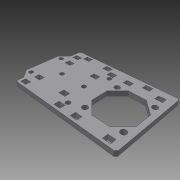
# Autodesk Inventor part: x_iddler_bottom
Saved by Autodesk Inventor 2014 (Build 180170000, 170)
## iProperties
Created: 2013-12-02
Part Number: x_iddler_bottom
Material: Generic
Document SubType Name: Modeling
Designer: buben
Density: 1 g/cm^3
Appearance: Default
Author: buben
Autodesk Inventor part; units mm, degrees
ref_plane "YZ Plane" through (0, 0, 0) normal (1, 0, 0) x (0, 1, 0)
ref_plane "XZ Plane" through (0, 0, 0) normal (0, 1, 0) x (-1, 0, 0)
ref_plane "XY Plane" through (0, 0, 0) normal (0, 0, 1) x (1, 0, 0)
sketch "Sketch1" plane through (0, 0, 0) normal (0, 0, 1) x (1, 0, 0)
  line L0 (0, 0) -> (-128, 0)
  line L1 (-128, 86) -> (0, 86)
  line L2 (0, 86) -> (0, 0)
  line L3 (-128, 71) -> (-138, 61)
  line L4 (-138, 61) -> (-138, 19)
  line L5 (-138, 19) -> (-128, 9)
  line L6 (-128, 0) -> (-128, 9)
  line L7 (-128, 71) -> (-128, 86)
  line L8 (-52, 9) -> (-44, 9)
  line L9 (-44, 9) -> (-44, 3)
  line L10 (-44, 3) -> (-52, 3)
  line L11 (-52, 3) -> (-52, 9)
  line L12 (-52, 77) -> (-44, 77)
  line L13 (-44, 77) -> (-44, 71)
  line L14 (-44, 71) -> (-52, 71)
  line L15 (-52, 71) -> (-52, 77)
  line L16 (-16, 77) -> (-8, 77)
  line L17 (-8, 77) -> (-8, 71)
  line L18 (-8, 71) -> (-16, 71)
  line L19 (-16, 71) -> (-16, 77)
  line L20 (-16, 9) -> (-8, 9)
  line L21 (-8, 9) -> (-8, 3)
  line L22 (-8, 3) -> (-16, 3)
  line L23 (-16, 3) -> (-16, 9)
  line L24 (-34, 83) -> (-26, 83)
  line L25 (-26, 83) -> (-26, 77)
  line L26 (-26, 77) -> (-34, 77)
  line L27 (-34, 77) -> (-34, 83)
  line L28 (-6, 49.9411) -> (-6, 30.0589)
  line L29 (-6, 30.0589) -> (-20.0589, 16)
  line L30 (-20.0589, 16) -> (-39.9411, 16)
  line L31 (-39.9411, 16) -> (-54, 30.0589)
  line L32 (-54, 30.0589) -> (-54, 49.9411)
  line L33 (-54, 49.9411) -> (-39.9411, 64)
  line L34 (-39.9411, 64) -> (-20.0589, 64)
  line L35 (-20.0589, 64) -> (-6, 49.9411)
  line L36 (-51, 61) -> (-9, 61) construction
  line L37 (-9, 61) -> (-9, 19) construction
  line L38 (-9, 19) -> (-51, 19) construction
  line L39 (-51, 19) -> (-51, 61) construction
  circle A0 centre (-51, 61) radius 3.2
  circle A1 centre (-51, 19) radius 3.2
  circle A2 centre (-9, 19) radius 3.2
  circle A3 centre (-9, 61) radius 3.2
  circle A4 centre (-131, 60) radius 2.75
  circle A5 centre (-131, 20) radius 2.75
  line L40 (-124, 77) -> (-116, 77)
  line L41 (-116, 77) -> (-116, 71)
  line L42 (-116, 71) -> (-124, 71)
  line L43 (-124, 71) -> (-124, 77)
  line L44 (-124, 9) -> (-116, 9)
  line L45 (-116, 9) -> (-116, 3)
  line L46 (-116, 3) -> (-124, 3)
  line L47 (-124, 3) -> (-124, 9)
  line L48 (-121, 63) -> (-113, 63)
  line L49 (-113, 63) -> (-113, 57)
  line L50 (-113, 57) -> (-121, 57)
  line L51 (-121, 57) -> (-121, 63)
  line L52 (-121, 23) -> (-113, 23)
  line L53 (-113, 23) -> (-113, 17)
  line L54 (-113, 17) -> (-121, 17)
  line L55 (-121, 17) -> (-121, 23)
  circle A6 centre (-66, 67) radius 2.75
  circle A7 centre (-66, 13) radius 2.75
  line L56 (-60, 86) -> (-60, 0) construction
  line L57 (-132, 67) -> (-60, 67) construction
  line L58 (-132, 13) -> (-60, 13) construction
  line L59 (-83, 63) -> (-75, 63)
  line L60 (-75, 63) -> (-75, 57)
  line L61 (-75, 57) -> (-83, 57)
  line L62 (-83, 57) -> (-83, 63)
  line L63 (-83, 23) -> (-75, 23)
  line L64 (-75, 23) -> (-75, 17)
  line L65 (-75, 17) -> (-83, 17)
  line L66 (-83, 17) -> (-83, 23)
  line L67 (-73, 77) -> (-65, 77)
  line L68 (-65, 77) -> (-65, 71)
  line L69 (-65, 71) -> (-73, 71)
  line L70 (-73, 71) -> (-73, 77)
  line L71 (-73, 9) -> (-65, 9)
  line L72 (-65, 9) -> (-65, 3)
  line L73 (-65, 3) -> (-73, 3)
  line L74 (-73, 3) -> (-73, 9)
  line L75 (-113, 83) -> (-105, 83)
  line L76 (-105, 83) -> (-105, 77)
  line L77 (-105, 77) -> (-113, 77)
  line L78 (-113, 77) -> (-113, 83)
  line L79 (-84, 83) -> (-76, 83)
  line L80 (-76, 83) -> (-76, 77)
  line L81 (-76, 77) -> (-84, 77)
  line L82 (-84, 77) -> (-84, 83)
  circle A8 centre (-106, 40) radius 2.75
  circle A9 centre (-74, 40) radius 2.75
  point P0 (-30, 40)
  point P1 (-138, 40)
  point P2 (-54, 40)
  point P3 (-51, 40)
  point P4 (-30, 61)
  point P5 (-30, 64)
  dimension "d1" = 45
  dimension "d2" = 10
  dimension "d3" = 6
  dimension "d4" = 6
  dimension "d5" = 3
  dimension "d6" = 8
  dimension "d7" = 8
  dimension "d8" = 6
  dimension "d10" = 3
  dimension "d11" = 48
  dimension "d12" = 8
  dimension "d13" = 6
  dimension "d14" = 42
  dimension "d15" = 42
  dimension "d16" = 6.4
  dimension "d17" = 6.4
  dimension "d18" = 6.4
  dimension "d19" = 6.4
  dimension "d20" = 5.5
  dimension "d21" = 5.5
  dimension "d22" = 7
  dimension "d23" = 11
  dimension "d24" = 11
  dimension "d25" = 6
  dimension "d26" = 8
  dimension "d27" = 6
  dimension "d28" = 6
  dimension "d29" = 8
  dimension "d30" = 6
  dimension "d31" = 8
  dimension "d32" = 8
  dimension "d33" = 5.5
  dimension "d34" = 5.5
  dimension "d35" = 4
  dimension "d36" = 4
  dimension "d37" = 8
  dimension "d38" = 8
  dimension "d39" = 8
  dimension "d40" = 4
  dimension "d41" = 8
  dimension "d42" = 128
  dimension "d43" = 68
  dimension "d44" = 8
  dimension "d45" = 43
  dimension "d47" = 10
  dimension "d48" = 15
  dimension "d49" = 62
  dimension "d50" = 10
  dimension "d52" = 8
  dimension "d53" = 3
  dimension "d54" = 8
  dimension "d55" = 3
  dimension "d56" = 5.5
  dimension "d57" = 5.5
  dimension "d58" = 14
  dimension "d59" = 32
  dimension "d65" = 34
  constraints: 166 end point, 37 parallel, 29 collinear, 21 perpendicular, 17 horizontal, 10 centre point, 9 horizontal alignment, 8 point on line, 5 midpoint, 4 coincident, 3 vertical alignment, 17 other
  measures "d1" angle of L7 L3
  measures "d2" distance between parallel lines of L7 L4
  measures "d3" distance of L16.end L17.end
  measures "d4" distance of L20.end L21.end
  measures "d5" distance between parallel lines of L0 L22
  measures "d6" distance of L16.start L16.end
  measures "d7" distance of L24.start L24.end
  measures "d8" distance of L24.end L25.end
  measures "d10" distance between parallel lines of L1 L24
  measures "d11" distance between parallel lines of L32 L28
  measures "d12" distance between parallel lines of L2 L17
  measures "d13" distance between parallel lines of L2 L28
  measures "d14" distance of L36.start L36.end
  measures "d15" distance of L38.end L36.start
  measures "d16" diameter of A0
  measures "d17" diameter of A3
  measures "d18" diameter of A1
  measures "d19" diameter of A2
  measures "d20" diameter of A5
  measures "d21" diameter of A4
  measures "d22" distance from line of L4 A4.centre
  measures "d23" vertical distance of A4.centre L3.start
  measures "d24" vertical distance of L5.end A5.centre
  measures "d25" distance of L42.end L40.start
  measures "d26" distance of L40.start L40.end
  measures "d27" distance of L46.end L44.start
  measures "d28" distance of L50.end L48.start
  measures "d29" distance of L48.start L48.end
  measures "d30" distance of L54.end L52.start
  measures "d31" distance between parallel lines of L42 L48
  measures "d32" distance between parallel lines of L44 L54
  measures "d33" diameter of A6
  measures "d34" diameter of A7
  measures "d35" distance between parallel lines of L58 L44
  measures "d36" distance between parallel lines of L57 L42
  measures "d37" distance of L59.start L59.end
  measures "d38" distance of L67.start L67.end
  measures "d39" distance of L72.end L73.end
  measures "d40" distance between parallel lines of L6 L47
  measures "d41" distance of L12.start L12.end
  measures "d42" distance of L0.start L0.end
  measures "d43" distance between parallel lines of L7 L56
  measures "d44" distance between parallel lines of L56 L15
  measures "d45" distance between parallel lines of L70 L41
  measures "d47" distance from line of L51 A4.centre
  measures "d48" distance between parallel lines of L56 L60
  measures "d49" distance from line of L7 A6.centre
  measures "d50" distance between parallel lines of L13 L27
  measures "d52" distance of L75.start L75.end
  measures "d53" distance between parallel lines of L41 L78
  measures "d54" distance of L79.start L79.end
  measures "d55" distance between parallel lines of L70 L80
  measures "d56" diameter of A8
  measures "d57" diameter of A9
  measures "d58" distance from line of L56 A9.centre
  measures "d59" distance from line of L4 A8.centre
  measures "d65" distance between parallel lines of L52 L50
extrude "Extrusion1" add sketch "Sketch1" along normal blind 6
chamfer "Chamfer1" distance 2 angle 45 4 edges at (-128, 0, 3) (-128, 86, 3) (0, 86, 3) (0, 0, 3)
body "Solid1"
